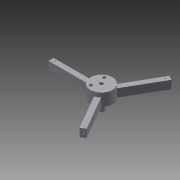
# Autodesk Inventor part: TriPost
Saved by Autodesk Inventor 2011 SP2 (Build 150309200, 309)
## iProperties
Created: 2013-02-08
Part Number: TriPost
Document SubType Name: Modeling
Designer: sungwook
Density: 2.71 g/cm^3
Material: Aluminum-6061
Mass: 3.84241 g
Surface Area: 15.4566 cm^2
Volume: 1.41786 cm^3
Author: sungwook
Autodesk Inventor part; units mm, degrees
ref_plane "YZ Plane" through (0, 0, 0) normal (1, 0, 0) x (0, 1, 0)
ref_plane "XZ Plane" through (0, 0, 0) normal (0, 1, 0) x (-1, 0, 0)
ref_plane "XY Plane" through (0, 0, 0) normal (0, 0, 1) x (1, 0, 0)
sketch "Sketch1" plane through (0, 0, 0) normal (0, 0, 1) x (1, 0, 0)
  circle A0 centre (0, 0) radius 5.461
  dimension "d0" = 10.922
  constraints: 1 centre point, 1 coincident
  measures "d0" diameter of A0
extrude "Extrusion1" add sketch "Sketch1" along normal blind 6.096
sketch "Sketch2" plane through (0, 0, 0) normal (0, 0, -1) x (-1, 0, 0)
  circle A0 centre (0, 0) radius 5.461 projected
  line L0 (0, -35) -> (0, 35) projected
  line L1 (35, 0) -> (-35, 0) projected
  line L2 (0, 1.27) -> (25, 1.27)
  line L3 (25, 1.27) -> (25, -1.27)
  line L4 (25, -1.27) -> (0, -1.27)
  line L5 (0, -1.27) -> (0, 1.27)
  line L6 (-1.0999, -0.635) -> (-13.5999, 21.0156)
  line L7 (-13.5999, 21.0156) -> (-11.4001, 22.2856)
  line L8 (-11.4001, 22.2856) -> (1.0999, 0.635)
  line L9 (1.0999, 0.635) -> (-1.0999, -0.635)
  line L10 (1.0999, -0.635) -> (-11.4001, -22.2856)
  line L11 (-11.4001, -22.2856) -> (-13.5999, -21.0156)
  line L12 (-13.5999, -21.0156) -> (-1.0999, 0.635)
  line L13 (-1.0999, 0.635) -> (1.0999, -0.635)
  circle A1 centre (0, 0) radius 25
  point P0 (25, 0)
  point P1 (-12.5, 21.6506)
  point P2 (-12.5, -21.6506)
  dimension "d3" = 2.54
  dimension "d6" = 360
  dimension "d8" = 50
  constraints: 24 end point, 3 tangent, 2 coincident, 2 parallel, 1 centre point, 1 horizontal, 1 horizontal alignment, 1 midpoint, 1 perpendicular, 1 point on line, 29 other
  measures "d3" distance between parallel lines of L4 L2
  measures "d8" diameter of A1
extrude "Extrusion2" add sketch "Sketch2" against normal blind 4 contours L1 L9 L8 L2 A0 | L1 A1 L4 A0 | A0 L2 A1 L1 | A0 L4 L10 L13 L1 | A1 L2 L3 | L3 L4 A1 | L13 L10 L4 L0 | L13 L12 L6 A0 L8 L0 | L9 L6 L1 | L0 L2 L8 L9 | L0 L10 A0 L12 L6 L9 | L1 L12 L13 | L2 L0 L8 | L10 L0 L4 | A0 L6 A1 L8 | L10 A1 L12 A0 | A1 L7 L8 | L10 L11 A1 | L6 L7 A1 | A1 L11 L12
sketch "Sketch6" plane through (0, 0, 0) normal (0, 0, -1) x (-1, 0, 0)
  line L0 (5.3113, 1.27) -> (25, 1.27) projected
  arc A0 (-3.7555, 3.9647) -> (-3.7555, -3.9647) centre (0, 0) ccw projected
  circle A1 centre (0, 0) radius 23.094
  line L1 (0, 0) -> (27, 0)
  line L2 (0, 0) -> (-13.5, -23.3827)
  line L3 (0, 0) -> (-13.5, 23.3827)
  point P0 (-11.547, 20)
  point P1 (23.094, 0)
  dimension "d26" = 360
  dimension "d28" = 40
  constraints: 6 end point, 3 coincident, 2 point on circle, 2 point on line, 1 centre point, 1 parallel, 8 other
  measures "d28" distance of A1.end A1.start
hole "Hole2" at (-23.094, 0, 0) direction (0, 0, 1) diameter 0.515 end through all
pattern_circular "Circular Pattern2" count 3 over 360 about axis through (0, 0, -10) along (0, 0, 1) of "Hole2"
sketch "Sketch8" plane through (11.4001, -22.2856, 0) normal (0.5, -0.8660254, 0) x (0.8660254, 0.5, 0)
  line L0 (2.54, 4) -> (0, 4) projected
  line L1 (1.27, -1.2192) -> (1.27, 7.3152) projected
  line L2 (1.27, 4) -> (1.27, 0)
  point P0 (1.27, 2)
  constraints: 2 end point, 2 midpoint, 1 collinear, 1 point on line
hole "Hole4" at (12.5, -21.6506, 2) direction (-0.5, 0.8660254, 0) diameter 1.181 depth 1.906 thread size "0-80 UNF" class "2B" standard "ANSI Unified Screw Threads"
pattern_circular "Circular Pattern3(Side_hole)" count 3 over 360 about axis through (0, 0, -10) along (0, 0, 1) of "Hole4"
sketch "Sketch18" plane through (0, 0, 6.096) normal (0, 0, 1) x (1, 0, 0)
  circle A0 centre (0, 0) radius 5.461 projected
  line L0 (-32.72, 0) -> (21.3198, 0) projected
  point P0 (3.81, 0)
  point P1 (-1.905, 3.2996)
  point P2 (-1.905, -3.2996)
  dimension "d87" = 3.81
  dimension "d90" = 360
  constraints: 1 point on line, 4 other
  measures "d87" distance of point (3.81, 0) A0.centre
hole "Hole7" at (-1.905, 3.2996, 6.096) at (-1.905, -3.2996, 6.096) direction (0, 0, -1) diameter 1.4732 end through all
sketch "Sketch22" plane through (0, 0, 0) normal (0, 0, -1) x (-1, 0, 0)
  arc A0 (-1.5558, -5.2347) -> (5.3113, -1.27) centre (0, 0) ccw projected
  circle A1 centre (0, 0) radius 1.4986
  dimension "d104" = 2.9972
  constraints: 1 centre point, 1 coincident
  measures "d104" diameter of A1
extrude "Extrusion9" add sketch "Sketch22" along normal blind 5.08
sketch "Sketch23" plane through (0, 0, 6.096) normal (0, 0, 1) x (1, 0, 0)
  circle A0 centre (0, 0) radius 5.461 projected
hole "Hole8" at (0, 0, 6.096) direction (0, 0, -1) diameter 1.778 end through all clearance for "Flat Head Machine Screw (82)" size "#0" standard "Ansi Unified Screw Threads"
body "Solid1"
